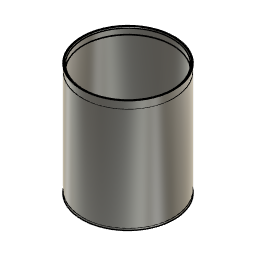
Lamp P3 (Autodesk Fusion 360 design; units mm, degrees)
Autodesk Fusion 360 part; units mm, degrees
sketch "Sketch1" plane through (0, 0, 0) normal (0, 0, 1) x (1, 0, 0)
  circle A0 centre (0, 0) radius 50
  constraint coincident A0.centre origin
extrude "Extrude1" add sketch "Sketch1" along normal blind 2
sketch "Sketch2" plane through (0, 0, 2) normal (0, 0, 1) x (-1, 0, 0)
  circle A0 centre (0, 0) radius 50
  circle A1 centre (0, 0) radius 49.5
  circle A2 centre (0, 0) radius 50
  dimension "d5" = 99
  constraint coincident A0.centre A1.centre
  measures "d5" diameter of A1
extrude "Extrude2" add sketch "Sketch2" along normal blind 120
sketch "Sketch3" plane through (0, 0, 122) normal (0, 0, 1) x (-1, 0, 0)
  circle A0 centre (0, 0) radius 49.5
  circle A1 centre (0, 0) radius 50
  circle A2 centre (0, 0) radius 48
  circle A3 centre (0, 0) radius 49.5
  constraint coincident A0.centre A1.centre
extrude "Extrude3" add sketch "Sketch3" against normal blind 8 contours A0 A3
chamfer "Chamfer1" distance 1 angle 45 2 edges at (44.7517, -17.3575, 122) (44.7517, 17.3575, 114)
